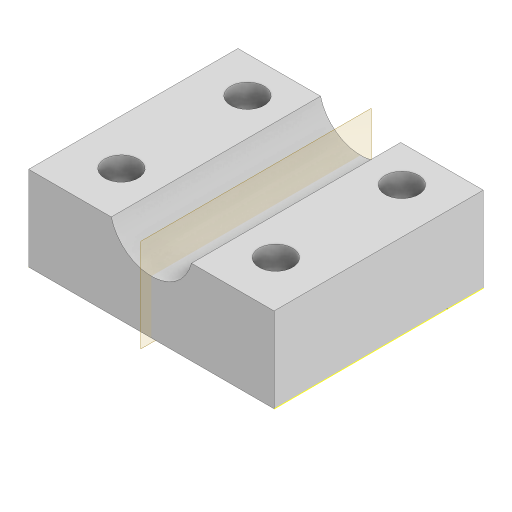
# Autodesk Inventor part: Нижняя часть крепления мотора
Saved by Autodesk Inventor 2023.2 (Build 272271030, 271C)
## iProperties
Created: 2024-12-16
Part Number: Нижняя часть крепления мотора
Material: Типовые
Document SubType Name: Modeling
Designer: I9232
Density: 1 g/cm^3
Appearance: По умолчанию
Author: I9232
Autodesk Inventor part; units mm, degrees
sketch "Эскиз1" plane through (0, 0, 0) normal (0, 1, 0) x (-1, 0, 0)
  line L0 (23.75, 20.25) -> (-23.75, 20.25)
  line L1 (-23.75, 20.25) -> (-23.75, -20.25)
  line L2 (-23.75, -20.25) -> (23.75, -20.25)
  line L3 (23.75, -20.25) -> (23.75, 20.25)
  line L4 (23.75, 20.25) -> (-23.75, -20.25) construction
  circle A0 centre (-15, 11.1546) radius 3.25
  line L5 (-0.0526, -1.582) -> (-0.0526, 1.3257) construction
  line L6 (1.5073, -1.0454) -> (-1.5235, -1.0454) construction
  circle A1 centre (14.8948, 11.1546) radius 3.25
  line L7 (-1.6126, -1.0454) -> (1.4182, -1.0454) construction
  circle A2 centre (-15, -13.2454) radius 3.25
  circle A3 centre (14.8948, -13.2454) radius 3.25
  line L8 (-15, 11.1546) -> (-23.75, 11.1546)
  line L9 (-15, 11.1546) -> (-15, 20.25)
  point P0 (0, 0)
  dimension "d0" = 47.5
  dimension "d1" = 40.5
  dimension "d6" = 6.5
  dimension "d10" = 8.75
  dimension "d11" = 9.0954
  constraints: 20 end point, 5 symmetric about line, 4 centre point, 3 perpendicular, 2 horizontal, 2 parallel, 2 point on line, 1 midpoint, 1 vertical, 3 other
  measures "d0" distance of L1.end L2.end
  measures "d1" distance of L0.end L1.end
  measures "d6" diameter of A3
  measures "d10" distance of L8.start L8.end
  measures "d11" distance of L8.start L9.end
extrude "Выдавливание1" add sketch "Эскиз1" along normal blind 16.4 contours L3 L2 L1 L8 A0 L9 L0 | L9 A0 L8 L1 L0
sketch "Эскиз2" plane through (-23.75, 0, 20.25) normal (0, 0, 1) x (1, 0, 0)
  line L0 (0, 0) -> (47.5, 0) projected
  line L1 (47.5, 0) -> (47.5, 16.4) projected
  line L2 (0, 16.4) -> (47.5, 16.4) projected
  line L3 (0, 0) -> (0, 16.4) projected
  line L4 (0, 0) -> (0, 16.4) projected
  line L5 (47.5, 0) -> (0, 0) projected
  line L6 (0, 16.4) -> (47.5, 0) construction
  line L7 (47.5, 16.4) -> (0, 16.4) projected
  line L8 (47.5, 16.4) -> (0, 0) construction
  arc A0 (15.9913, 16.4) -> (31.5087, 16.4) centre (23.75, 18.35) ccw
  line L9 (23.75, 8.2) -> (23.75, 18.35) construction
  point P0 (23.75, 0)
  point P1 (15.9913, 16.4)
  dimension "d15" = 1.95
  dimension "d16" = 16
  constraints: 6 end point, 2 point on circle, 2 point on line, 1 centre point, 1 coincident, 1 midpoint, 1 vertical
  measures "d15" distance from line of L2 A0.centre
  measures "d16" diameter of A0
extrude "Выдавливание4" cut sketch "Эскиз2" against normal up to surface (40.5 mm away) contours L2 A0
sketch "Эскиз3" plane through (0, 0, 0) normal (0, -1, 0) x (1, 0, 0)
  line L0 (23.75, -13.2454) -> (-23.75, -13.2454)
  line L1 (-23.75, -20.25) -> (-23.75, 20.25) projected
  line L2 (23.75, 20.25) -> (23.75, -20.25) projected
  circle A0 centre (15, -13.2454) radius 3.25 projected
  point P0 (0, 0)
  constraints: 3 point on line, 2 end point, 1 horizontal
ref_plane "РабПлоскость2" through (0, 0, 20.25) normal (1, 0, 0) x (0, 0, -1)
